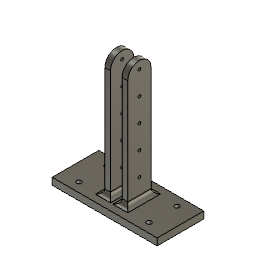
MAE148_Titlted_Camera (Autodesk Fusion 360 design; units mm, degrees)
part number: 2026-08-11-20-06-07-962
Autodesk Fusion 360 part; units mm, degrees
sketch "Sketch1" plane through (0, 0, 0) normal (0, 0, 1) x (1, 0, 0)
  line L0 (0, 0) -> (114.3, 0)
  line L1 (114.3, 0) -> (114.3, 50.8)
  line L2 (114.3, 50.8) -> (0, 50.8)
  line L3 (0, 50.8) -> (0, 0)
  point P0 (114.3, 25.4)
  point P1 (57.15, 0)
  dimension "d1" = 114.3
  dimension "d4" = 50.8
  constraint horizontal L0
  constraint vertical L1
  constraint horizontal L2
  constraint vertical L3
  constraint coincident L0.start L3.end
  constraint midpoint L1 P0
  constraint midpoint L0 P1
  measures "d1" distance of L1 L3
  measures "d4" distance of L0 L2
extrude "Extrude4" add sketch "Sketch1" along normal blind 7.62
sketch "Sketch2" plane through (0, 0, 7.62) normal (0, 0, 1) x (-1, 0, 0)
  line L0 (0, -50.8) -> (0, 0)
  line L1 (0, 0) -> (-114.3, 0)
  line L2 (-114.3, 0) -> (-114.3, -50.8)
  line L3 (-114.3, -50.8) -> (0, -50.8)
  line L4 (-44.704, -38.1) -> (-69.596, -38.1)
  line L5 (-69.596, -38.1) -> (-69.596, -12.7)
  line L6 (-69.596, -12.7) -> (-44.704, -12.7)
  line L7 (-44.704, -12.7) -> (-44.704, -38.1)
  line L8 (-63.5, -38.1) -> (-50.8, -38.1)
  line L9 (-50.8, -38.1) -> (-50.8, -12.7)
  line L10 (-50.8, -12.7) -> (-63.5, -12.7)
  line L11 (-63.5, -12.7) -> (-63.5, -38.1)
  line L12 (-63.5, -38.1) -> (-50.8, -12.7) construction
  line L13 (-50.8, -38.1) -> (-63.5, -12.7) construction
  circle A0 centre (-19.05, -40.64) radius 2.5
  line L14 (-57.15, -50.8) -> (-57.15, 0) construction
  line L15 (0, -25.4) -> (-114.3, -25.4) construction
  circle A1 centre (-95.25, -40.64) radius 2.5
  circle A2 centre (-19.05, -10.16) radius 2.5
  circle A3 centre (-95.25, -10.16) radius 2.5
  point P0 (-57.15, -38.1)
  point P1 (-69.596, -25.4)
  point P2 (-114.3, -25.4)
  point P3 (-57.15, 0)
  point P4 (-57.15, -25.4)
  dimension "d15" = 25.4
  dimension "d23" = 12.7
  dimension "d24" = 5
  dimension "d25" = 76.2
  dimension "d26" = 30.48
  dimension "d27" = 15.24
  dimension "d43" = 6.096
  dimension "d45" = 6.096
  constraint horizontal L4
  constraint vertical L5
  constraint horizontal L6
  constraint vertical L7
  constraint midpoint L4 P0
  constraint midpoint L5 P1
  constraint horizontal P1 P2
  constraint vertical P0 P3
  constraint horizontal L8
  constraint perpendicular L8 L9
  constraint parallel L8 L10
  constraint parallel L9 L11
  constraint coincident L12 P4
  constraint coincident L13 P4
  constraint coincident L4 L8.start
  constraint collinear L6 L10
  constraint midpoint L3 L14.start
  constraint coincident P3 L14.end
  constraint midpoint L0 L15.start
  constraint coincident P2 L15.end
  constraint symmetric A0 L14 A1
  constraint symmetric A0 L15 A2
  constraint symmetric L15 A1 A3
  measures "d15" distance of L4 L6
  measures "d23" distance of L9 L11
  measures "d24" diameter of A0
  measures "d25" distance of A0.centre A1.centre
  measures "d26" distance of A0.centre A2.centre
  measures "d27" distance of A0.centre L15
  measures "d43" distance of L7 L9
  measures "d45" distance of L5 L11
extrude "Extrude5" add sketch "Sketch2" along normal blind 132.08 contours L4 L6 L7 L9 | L4 L5 L6 L11
sketch "Sketch3" plane through (69.596, 0, 0) normal (1, 0, 0) x (0, 1, 0)
  line L0 (12.7, 7.62) -> (38.1, 7.62)
  line L1 (38.1, 7.62) -> (38.1, 139.7)
  line L2 (38.1, 139.7) -> (12.7, 139.7)
  line L3 (12.7, 139.7) -> (12.7, 7.62)
  circle A0 centre (25.4, 131.3981) radius 1.5
  circle A1 centre (25.4, 105.9981) radius 1.4986
  line L4 (25.4, 7.62) -> (25.4, 27.94) construction
  circle A2 centre (25.4, 80.5981) radius 1.4986
  circle A3 centre (25.4, 55.1981) radius 1.4986
  circle A4 centre (25.4, 29.7981) radius 1.4986
  point P0 (25.4, 139.7)
  dimension "d19" = 3
  dimension "d20" = 2.9972
  dimension "d21" = 25.4
  dimension "d37" = 2.9972
  dimension "d38" = 2.9972
  dimension "d39" = 2.9972
  dimension "d40" = 25.4
  dimension "d41" = 25.4
  dimension "d42" = 25.4
  constraint midpoint L2 P0
  constraint vertical A0.centre P0
  constraint vertical A0.centre A1.centre
  constraint midpoint L0 L4.start
  constraint perpendicular L0 L4
  constraint vertical A1.centre A2.centre
  constraint vertical A1.centre A3.centre
  constraint vertical A1.centre A4.centre
  measures "d19" diameter of A0
  measures "d20" diameter of A1
  measures "d21" distance of A0.centre A1.centre
  measures "d37" diameter of A2
  measures "d38" diameter of A3
  measures "d39" diameter of A4
  measures "d40" distance of A1.centre A2.centre
  measures "d41" distance of A2.centre A3.centre
  measures "d42" distance of A3.centre A4.centre
extrude "Extrude6" cut sketch "Sketch3" against normal through all contours A0 | A1 | A2 | A3 | A4
extrude "Extrude7" cut sketch "Sketch2" against normal through all contours A0 | A1 | A2 | A3
fillet "Fillet9" radius 12.7 4 edges at (66.548, 12.7, 139.7) (47.752, 12.7, 139.7) (47.752, 38.1, 139.7) (66.548, 38.1, 139.7)
fillet "Fillet10" radius 5.08 8 edges at (69.596, 25.4, 7.62) (66.548, 38.1, 7.62) (63.5, 25.4, 7.62) (44.704, 25.4, 7.62) (47.752, 38.1, 7.62) (50.8, 25.4, 7.62) (47.752, 12.7, 7.62) (66.548, 12.7, 7.62)
equation "d37 = d20"
equation "d38 = d20"
equation "d39 = d20"
equation "d45 = d43"
